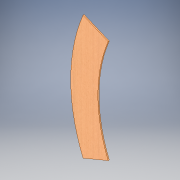
# Autodesk Inventor part: rearformer1
Saved by Autodesk Inventor 2019 (Build 230136000, 136)
## iProperties
Created: 2019-01-07
Part Number: rearformer1
Material: Wood (Cherry)
Document SubType Name: Modeling
Designer: gaincarlo
Density: 0.63 g/cm^3
Appearance: Cherry - Natural Low Gloss
Author: gaincarlo
Autodesk Inventor part; units mm, degrees
ref_plane "YZ Plane" through (0, 0, 0) normal (1, 0, 0) x (0, 1, 0)
ref_plane "XZ Plane" through (0, 0, 0) normal (0, 1, 0) x (-1, 0, 0)
ref_plane "Work Plane1" through (0, 0, 0) normal (0, 0, 1) x (1, 0, 0)
sketch "Sketch1" plane through (0, 0, 0) normal (0, 0, 1) x (1, 0, 0)
  line L0 (-254.3277, 283.4578) -> (-250.5009, 292.6966) construction
  line L1 (-250.5009, 292.6966) -> (303.8268, 63.0866) construction
  line L2 (303.8268, 63.0866) -> (300, 53.8478) construction
  line L3 (300, 53.8478) -> (-254.3277, 283.4578) construction
  line L4 (300, -53.8478) -> (303.8268, -63.0866) construction
  line L5 (303.8268, -63.0866) -> (-250.5009, -292.6966) construction
  line L6 (-250.5009, -292.6966) -> (-254.3277, -283.4578) construction
  line L7 (-254.3277, -283.4578) -> (300, -53.8478) construction
  arc A0 (-26.405, 186.8763) -> (-26.405, -186.8763) centre (430, 0) ccw construction
  spline S0 degree 3 poles (-26.405, -186.8763) (-26.7438, -187.0153) (-27.0825, -187.1543) (-27.76, -187.4323) (-28.0988, -187.5712) (-28.4375, -187.7102) knots -0.219692 -0.219692 -0.219692 -0.219692 -0.109846 -0.109846 0 0 0 0 construction
  arc A1 (-28.4375, 187.7102) -> (-28.4375, -187.7102) centre (430, 0) ccw construction
  spline S1 degree 3 poles (-28.4375, 187.7102) (-28.0988, 187.5712) (-27.76, 187.4323) (-27.0825, 187.1543) (-26.7438, 187.0153) (-26.405, 186.8763) knots -0.219692 -0.219692 -0.219692 -0.219692 -0.109846 -0.109846 0 0 0 0 construction
  line L8 (-27.6703, -189.5732) -> (-120, -227.8175)
  line L9 (-27.6703, 189.5732) -> (-120, 227.8175)
  arc A2 (-27.6703, 189.5732) -> (-27.6703, -189.5732) centre (430, 0) ccw
  arc A3 (-120, 227.8175) -> (-120, -227.8175) centre (430, 0) ccw
  point P0 (0, 0)
  dimension "d3" = 99.937
  constraints: 20 end point, 8 point on circle, 4 centre point, 4 point on line, 2 coincident, 30 other
  measures "d3" radial gap between concentric circles of A1 A3
extrude "Extrusion1" add sketch "Sketch1" against normal blind 4
body "Solid1"
